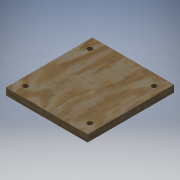
# Autodesk Inventor part: miniplatv3
Saved by Autodesk Inventor 2017 (Build 210142000, 142)
## iProperties
Created: 2016-04-30
Part Number: miniplatv3
Material: Wood (Oak)
Document SubType Name: Modeling
Designer: ypatel4
Density: 0.76 g/cm^3
Appearance: White Oak - Natural Medium Gloss
Mass: 622.478 g
Surface Area: 1103.24 cm^2
Volume: 819.05 cm^3
Author: ypatel4
Autodesk Inventor part; units mm, degrees
ref_plane "YZ Plane" through (0, 0, 0) normal (1, 0, 0) x (0, 1, 0)
ref_plane "Work Plane1" through (0, 25.4, 0) normal (0, 1, 0) x (1, 0, 0)
sketch "Sketch3" plane through (0, 25.4, 0) normal (0, 1, 0) x (1, 0, 0)
  line L0 (-104.775, -111.125) -> (104.775, -111.125)
  line L1 (104.775, -111.125) -> (104.775, 111.125)
  line L2 (104.775, 111.125) -> (-104.775, 111.125)
  line L3 (-104.775, 111.125) -> (-104.775, -111.125)
  line L4 (-104.775, -111.125) -> (104.775, 111.125) construction
  line L5 (104.775, -111.125) -> (-104.775, 111.125) construction
  point P0 (0, 0)
  dimension "d13" = 209.55
  dimension "d14" = 222.25
  constraints: 12 end point, 2 midpoint, 2 parallel, 1 horizontal, 1 perpendicular
  measures "d13" distance of L2.end L1.end
  measures "d14" distance of L1.end L0.end
ref_plane "Work Plane2" through (-90.8689, 50.8, 86.2283) normal (0, 1, 0) x (1, 0, 0)
sketch "Sketch4" plane through (-90.8689, 50.8, 86.2283) normal (0, 1, 0) x (1, 0, 0)
  line L0 (-13.9061, -24.8967) -> (195.6439, -24.8967)
  line L1 (195.6439, -24.8967) -> (195.6439, 197.3533)
  line L2 (195.6439, 197.3533) -> (-13.9061, 197.3533)
  line L3 (-13.9061, 197.3533) -> (-13.9061, -24.8967)
  line L4 (-13.9061, -24.8967) -> (195.6439, 197.3533) construction
  line L5 (195.6439, -24.8967) -> (-13.9061, 197.3533) construction
  point P0 (90.8689, 86.2283)
  point P1 (90.8689, 86.2283)
  dimension "d15" = 209.55
  dimension "d16" = 222.25
  constraints: 12 end point, 2 midpoint, 2 parallel, 1 coincident, 1 horizontal, 1 perpendicular
  measures "d15" distance of L2.end L1.end
  measures "d16" distance of L1.end L0.end
extrude "Extrusion2" add sketch "Sketch4" along normal blind 17.78
sketch "Sketch6" plane through (-90.8689, 68.58, 86.2283) normal (0, 1, 0) x (1, 0, 0)
  line L0 (173.5232, 168.8826) -> (8.2147, 168.8826) construction
  line L1 (8.2147, 3.5741) -> (8.2147, 168.8826) construction
  line L2 (173.5232, 168.8826) -> (173.5232, 3.5741) construction
  circle A0 centre (8.2147, 168.8826) radius 6.35
  circle A1 centre (173.5232, 168.8826) radius 6.35
  circle A2 centre (173.5232, 3.5741) radius 6.35
  circle A3 centre (8.2147, 3.5741) radius 6.35
  point P0 (90.8689, 86.2283)
  dimension "d33" = 12.7
  dimension "d34" = 12.7
  dimension "d35" = 12.7
  dimension "d36" = 12.7
  constraints: 6 end point, 4 centre point, 4 coincident, 1 vertical
  measures "d33" diameter of A0
  measures "d34" diameter of A1
  measures "d35" diameter of A2
  measures "d36" diameter of A3
hole "Hole2" at (-82.6543, 68.58, -82.6543) at (82.6543, 68.58, -82.6543) at (82.6543, 68.58, 82.6543) at (-82.6543, 68.58, 82.6543) direction (0, -1, 0) diameter 12.7 end through all
body "Solid1"
